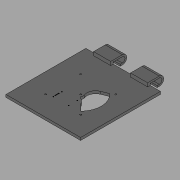
# Autodesk Inventor part: bin_lid
Saved by Autodesk Inventor 2019 (Build 230136000, 136)
## iProperties
Part Number: bin_lid
Material: Generic
Document SubType Name: Modeling
Designer: Javi
Appearance: Default
Author: Javi
Autodesk Inventor part; units mm, degrees
ref_plane "YZ Plane" through (0, 0, 0) normal (1, 0, 0) x (0, 1, 0)
ref_plane "XZ Plane" through (0, 0, 0) normal (0, 1, 0) x (-1, 0, 0)
ref_plane "XY Plane" through (0, 0, 0) normal (0, 0, 1) x (1, 0, 0)
sketch "Sketch6" plane through (0, 0, 0) normal (0, 1, 0) x (-1, 0, 0)
  line L0 (0, 0) -> (-436, 0)
  line L1 (-436, 0) -> (-436, -467)
  line L2 (-436, -467) -> (0, -467)
  line L3 (0, -467) -> (0, 0)
  dimension "d25" = 436
  dimension "d26" = 467
  constraints: 8 end point, 2 parallel, 1 horizontal, 1 perpendicular
  measures "d25" distance of L2.end L1.end
  measures "d26" distance of L1.end L0.end
extrude "Extrusion5" add sketch "Sketch6" along normal blind 56
sketch "Sketch7" plane through (436, 0, -467) normal (0, 0, -1) x (-1, 0, 0)
  line L0 (436, 0) -> (0, 0) projected
  line L1 (218, 0) -> (376, 0)
  line L2 (218, 0) -> (376, 0) construction
  line L3 (376, 0) -> (376, 56)
  line L4 (436, 56) -> (0, 56) projected
  line L5 (376, 56) -> (60, 56)
  line L6 (376, 56) -> (692, 56) construction
  line L7 (60, 56) -> (60, 0)
  line L8 (60, 0) -> (218, 0)
  line L9 (60, 0) -> (160, 0)
  line L10 (160, 0) -> (160, 56)
  line L11 (376, 0) -> (276, 0)
  line L12 (376, 0) -> (476, 0) construction
  line L13 (276, 0) -> (276, 56)
  dimension "d29" = 158
  dimension "d30" = 0
  dimension "d31" = 316
  dimension "d32" = 180
  dimension "d33" = 100
  dimension "d34" = 100
  dimension "d35" = 180
  constraints: 24 end point, 6 perpendicular, 5 collinear, 5 point on line, 3 horizontal, 1 midpoint
  measures "d29" distance of L1.start L1.end
  measures "d30" distance between parallel lines of L1 L2
  measures "d31" distance of L3.end L5.end
  measures "d32" angle of L5 L6
  measures "d33" distance of L7.end L9.end
  measures "d34" distance of L1.end L11.end
  measures "d35" angle of L11 L12
extrude "Extrusion6" add sketch "Sketch7" along normal blind 100 contours L0 L13 L4 L3 | L0 L7 L4 L10
sketch "Sketch8" plane through (0, 0, -467) normal (-1, 0, 0) x (0, 0, 1)
  arc A0 (-53, 44) -> (-53, 12) centre (-53, 28) ccw
  line L0 (0, 0) -> (-100, 0) projected
  line L1 (-100, 0) -> (-100, 56) projected
  arc A1 (-53, 54) -> (-53, 2) centre (-53, 28) ccw
  line L2 (0, 0) -> (-100, 0)
  line L3 (-100, 56) -> (-100, 0) projected
  line L4 (-100, 0) -> (-100, 56)
  line L5 (0, 56) -> (-100, 56) projected
  line L6 (-100, 56) -> (0, 56)
  line L7 (-53, 54) -> (0, 54)
  line L8 (-53, 12) -> (-40, 12)
  line L9 (-40, 12) -> (-40, 2)
  line L10 (-40, 2) -> (-53, 2)
  line L11 (-53, 44) -> (0, 44)
  line L12 (467, 0) -> (0, 0) projected
  line L13 (0, 56) -> (0, 0)
  line L14 (0, 44) -> (0, 54)
  point P0 (467, 56)
  dimension "d30" = 0
  dimension "d32" = 180
  dimension "d35" = 180
  dimension "d38" = 28
  dimension "d39" = 32
  dimension "d40" = 47
  dimension "d45" = 52
  dimension "d50" = 13
  constraints: 20 end point, 4 point on circle, 4 tangent, 3 horizontal, 2 centre point, 2 collinear, 2 perpendicular, 2 vertical, 1 coincident, 1 parallel
  measures "d38" distance from line of L0 A0.centre
  measures "d39" diameter of A0
  measures "d40" distance from line of L1 A0.centre
  measures "d45" diameter of A1
  measures "d50" distance of L8.start L8.end
extrude "Extrusion8" cut sketch "Sketch8" against normal through all contours L11 L13 L0 L1 L5 L7 A1 L10 L9 L8 A0
sketch "Sketch9" plane through (0, 0, -467) normal (-1, 0, 0) x (0, 0, 1)
  line L0 (467, 0) -> (0, 0) projected
  line L1 (0, 0) -> (467, 0)
  line L2 (467, 0) -> (467, 18)
  line L3 (467, 18) -> (0, 18)
  line L4 (0, 18) -> (0, 0)
  line L5 (0, 0) -> (0, 56) projected
  line L6 (467, 0) -> (467, 56) projected
  line L7 (0, 56) -> (467, 56)
  line L8 (467, 56) -> (467, 54)
  line L9 (467, 54) -> (0, 54)
  line L10 (0, 54) -> (0, 56)
  dimension "d59" = 467
  dimension "d60" = 18
  dimension "d61" = 2
  constraints: 16 end point, 4 parallel, 2 horizontal, 2 perpendicular, 1 point on line
  measures "d59" distance of L3.end L2.end
  measures "d60" distance of L2.end L1.end
  measures "d61" distance of L7.end L8.end
extrude "Extrusion9" cut sketch "Sketch9" against normal through all contours L0 L4 L3 L2 | L9 L5 L7 L6
sketch "Sketch10" plane through (0, 54, 0) normal (0, 1, 0) x (1, 0, 0)
  line L0 (376, 520) -> (376, 467) projected
  line L1 (436, 467) -> (436, 0) projected
  line L2 (376, 467) -> (436, 467)
  line L3 (436, 467) -> (436, 0)
  line L4 (436, 0) -> (0, 0) projected
  line L5 (436, 0) -> (0, 0)
  line L6 (0, 467) -> (60, 467) projected
  line L7 (0, 0) -> (0, 467)
  line L8 (0, 467) -> (60, 467)
  line L9 (60, 467) -> (60, 452)
  line L10 (60, 452) -> (160, 452)
  line L11 (160, 520) -> (160, 467) projected
  line L12 (160, 452) -> (160, 467)
  line L13 (276, 467) -> (276, 520) projected
  line L14 (160, 467) -> (276, 467)
  line L15 (276, 467) -> (276, 452)
  line L16 (276, 452) -> (376, 452)
  line L17 (376, 452) -> (376, 467)
  dimension "d64" = 15
  dimension "d65" = 90
  constraints: 24 end point, 7 perpendicular, 4 collinear, 1 horizontal, 1 point on line
  measures "d64" distance of L6.end L9.end
  measures "d65" angle of L8 L9
extrude "Extrusion10" cut sketch "Sketch10" against normal blind 21
sketch "Sketch11" plane through (0, 33, 0) normal (0, 1, 0) x (1, 0, 0)
  circle A0 centre (218, 218.5) radius 4.25
  line L0 (0, 0) -> (0, 467) projected
  line L1 (436, 0) -> (0, 0) projected
  dimension "d70" = 8.5
  dimension "d71" = 218
  dimension "d72" = 218.5
  constraints: 1 centre point
  measures "d70" diameter of A0
  measures "d71" distance from line of L0 A0.centre
  measures "d72" distance from line of L1 A0.centre
extrude "Extrusion11" cut sketch "Sketch11" against normal through all
sketch "Sketch12" plane through (0, 33, 0) normal (0, 1, 0) x (1, 0, 0)
  circle A0 centre (218, 218.5) radius 4.25 projected
  circle A1 centre (218, 218.5) radius 120
  circle A2 centre (218, 218.5) radius 15
  line L0 (231.9078, 224.1191) -> (329.2621, 263.4528)
  line L1 (233, 218.5) -> (338, 218.5)
  arc A3 (329.2621, 263.4528) -> (231.9078, 224.1191) centre (280.5849, 243.7859) ccw
  circle A4 centre (218, 218.5) radius 145
  circle A5 centre (320.5305, 115.9695) radius 4.5
  circle A6 centre (320.5305, 321.0305) radius 4.5
  circle A7 centre (115.4695, 321.0305) radius 4.5
  circle A8 centre (115.4695, 115.9695) radius 4.5
  line L2 (320.5305, 115.9695) -> (302.8528, 133.6472)
  line L3 (320.5305, 115.9695) -> (345.5305, 115.9695) construction
  line L4 (222.25, 218.5) -> (233, 218.5)
  line L5 (218, 203.5) -> (218, 150.5)
  line L6 (218, 218.5) -> (281, 218.5) construction
  arc A9 (266, 170.5) -> (238, 198.5) centre (218, 150.5) ccw
  line L7 (302.8528, 133.6472) -> (266, 170.5)
  line L8 (238, 198.5) -> (228.6066, 207.8934)
  line L9 (218, 203.5) -> (218, 214.25)
  line L10 (260.9181, 292.4631) -> (298.382, 307.5995)
  point P0 (0, 0)
  dimension "d81" = 290
  dimension "d76" = 30
  dimension "d77" = 240
  dimension "d82" = 9
  dimension "d87" = 360
  dimension "d90" = 135
  dimension "d91" = 22
  dimension "d92" = 68
  dimension "d95" = 52
  constraints: 22 end point, 15 point on circle, 8 centre point, 7 line through centre, 4 coincident, 4 horizontal, 2 tangent, 2 vertical, 1 equal length, 1 point on line, 12 other
  measures "d76" diameter of A2
  measures "d77" diameter of A1
  measures "d82" diameter of A5
  measures "d90" angle of L3 L2
  measures "d91" angle of L4 L0
  measures "d92" distance of L6.start L5.end
  measures "d95" radius of A9
extrude "Extrusion12" cut sketch "Sketch12" against normal through all contours L1 A1 L7 A9 L8 A2 | A2 L0 A1 L1 | A3 L0 | A3 L10 A1 | A6 A4 | A4 A6 | A5 A4 | A4 L2 A5 | A4 A5 L2 | A7 A4 | A4 A7 | A8 A4 | A4 A8
sketch "Sketch13" plane through (0, 18, -467) normal (0, -1, 0) x (1, 0, 0)
  arc A0 (179.5346, 284.9654) -> (179.5346, 344.9654) centre (219.5346, 314.9654) ccw
  line L0 (144.5346, 344.9654) -> (244.5346, 344.9654)
  line L1 (244.5346, 344.9654) -> (244.5346, 284.9654)
  line L2 (244.5346, 284.9654) -> (144.5346, 284.9654)
  line L3 (144.5346, 284.9654) -> (144.5346, 344.9654)
  point P0 (0, 467)
  point P1 (266, 296.5)
  point P2 (238, 268.5)
  dimension "d96" = 100
  dimension "d97" = 100
  dimension "d98" = 60
  dimension "d99" = 25
  dimension "d100" = 30
  constraints: 8 end point, 4 point on circle, 2 parallel, 2 point on line, 1 centre point, 1 horizontal, 1 perpendicular
  measures "d96" diameter of A0
  measures "d97" distance of L1.end L2.end
  measures "d98" distance of L0.end L1.end
  measures "d99" distance from line of A0.centre L1
  measures "d100" distance from line of L2 A0.centre
extrude "Extrusion13" cut sketch "Sketch13" against normal blind 13 contours L2 L3 L0 L1
sketch "Sketch14" plane through (0, 31, -467) normal (0, -1, 0) x (1, 0, 0)
  line L0 (144.5346, 284.9654) -> (144.5346, 344.9654) projected
  line L1 (244.5346, 284.9654) -> (144.5346, 284.9654) projected
  line L2 (244.5346, 344.9654) -> (244.5346, 284.9654) projected
  line L3 (144.5346, 344.9654) -> (244.5346, 344.9654) projected
  circle A0 centre (239.5346, 289.9654) radius 1.75
  circle A1 centre (149.5346, 289.9654) radius 1.75
  circle A2 centre (239.5346, 339.9654) radius 1.75
  circle A3 centre (149.5346, 339.9654) radius 1.75
  line L4 (147.0346, 329.9654) -> (151.0346, 329.9654)
  line L5 (151.0346, 329.9654) -> (151.0346, 304.9654)
  line L6 (151.0346, 304.9654) -> (147.0346, 304.9654)
  line L7 (147.0346, 304.9654) -> (147.0346, 329.9654)
  point P0 (0, 467)
  dimension "d103" = 3.5
  dimension "d104" = 5
  dimension "d105" = 5
  dimension "d108" = 90
  dimension "d111" = 50
  dimension "d117" = 4
  dimension "d118" = 25
  dimension "d119" = 15
  dimension "d120" = 2.5
  constraints: 8 end point, 4 centre point, 2 horizontal, 2 parallel, 1 perpendicular, 1 vertical, 6 other
  measures "d103" diameter of A0
  measures "d104" distance from line of L1 A0.centre
  measures "d105" distance from line of A0.centre L2
  measures "d108" distance of A0.centre A1.centre
  measures "d111" distance of A0.centre A2.centre
  measures "d117" distance of L5.end L6.end
  measures "d118" distance of L4.end L5.end
  measures "d119" distance between parallel lines of L3 L4
  measures "d120" distance between parallel lines of L0 L7
extrude "Extrusion14" cut sketch "Sketch14" against normal through all contours A0 | A1 | A2 | A3 | L4 L5 L6 L7
chamfer "Chamfer1" distance 1 angle 45 4 edges at (147.7846, 33, -177.0346) (147.7846, 33, -127.0346) (237.7846, 33, -127.0346) (237.7846, 33, -177.0346)
body "Solid2"
